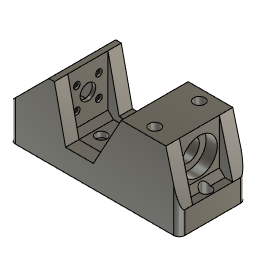
Stepper Motor Mount Mk4 Long v11 (Autodesk Fusion 360 design; units mm, degrees)
Autodesk Fusion 360 part; units mm, degrees
sketch "Sketch1" plane through (0, 0, 0) normal (0, 0, 1) x (1, 0, 0)
  line L0 (0, 0) -> (152, 0)
  line L1 (152, 0) -> (152, 60)
  line L2 (152, 60) -> (0, 60)
  line L3 (0, 60) -> (0, 0)
  dimension "d1" = 152
  dimension "d2" = 60
  constraint horizontal L0
  constraint vertical L1
  constraint horizontal L2
  constraint vertical L3
  constraint coincident L0.start L3.end
  measures "d1" distance of L0.start L0.end
  measures "d2" distance of L0.start L2.end
extrude "Extrude1" add sketch "Sketch1" along normal blind 10
sketch "Sketch2" plane through (0, 0, 10) normal (0, 0, 1) x (-1, 0, 0)
  line L0 (0, -60) -> (0, 0)
  line L1 (0, 0) -> (-152, 0)
  line L2 (-152, 0) -> (-152, -60)
  line L3 (-152, -60) -> (0, -60)
  line L4 (-35, -60) -> (-40, -60)
  line L5 (-40, -60) -> (-40, 0)
  line L6 (-40, 0) -> (-35, 0)
  line L7 (-35, 0) -> (-35, -60)
  line L8 (-140, -60) -> (-100, -60)
  line L9 (-100, -60) -> (-100, 0)
  line L10 (-100, 0) -> (-140, 0)
  line L11 (-140, 0) -> (-140, -60)
  dimension "d5" = 5
  dimension "d6" = 35
  dimension "d25" = 40
  dimension "d91" = 12
  constraint horizontal L4
  constraint vertical L5
  constraint horizontal L6
  constraint vertical L7
  constraint coincident L3 L4.start
  constraint horizontal L8
  constraint vertical L9
  constraint horizontal L10
  constraint vertical L11
  constraint coincident L1 L9.end
  constraint collinear L3 L8
  measures "d5" distance of L4.start L4.end
  measures "d6" distance of L0 L7
  measures "d25" distance of L9 L11
  measures "d91" distance of L2 L11
extrude "Extrude2" add sketch "Sketch2" along normal blind 56 contours L1 L3 L4 L5 L6 L7 | L1 L3 L8 L9 L10 L11
sketch "Sketch3" plane through (40, 0, 0) normal (1, 0, 0) x (0, 1, 0)
  line L0 (0, 10) -> (60, 10)
  line L1 (60, 10) -> (60, 66)
  line L2 (60, 66) -> (0, 66)
  line L3 (0, 66) -> (0, 10)
  circle A0 centre (30, 43) radius 14 construction
  circle A1 centre (20.1005, 52.8995) radius 1.6
  circle A2 centre (39.8995, 52.8995) radius 1.6
  circle A3 centre (20.1005, 33.1005) radius 1.6
  circle A4 centre (39.8995, 33.1005) radius 1.6
  line L4 (30, 43) -> (39.8995, 33.1005) construction
  line L5 (30, 43) -> (45, 43) construction
  line L6 (30, 43) -> (20.1005, 33.1005) construction
  line L7 (30, 43) -> (45, 43) construction
  line L8 (30, 43) -> (20.1005, 52.8995) construction
  line L9 (30, 43) -> (45, 43) construction
  line L10 (30, 43) -> (39.8995, 52.8995) construction
  line L11 (30, 43) -> (45, 43) construction
  circle A5 centre (30, 43) radius 7
  dimension "d9" = 28
  dimension "d10" = 30
  dimension "d11" = 3.2
  dimension "d12" = 3.2
  dimension "d13" = 3.2
  dimension "d14" = 3.2
  dimension "d17" = 33
  dimension "d18" = 45
  dimension "d19" = 135
  dimension "d20" = 135
  dimension "d21" = 45
  dimension "d24" = 14
  constraint coincident A0 A1.centre
  constraint coincident A0 A2.centre
  constraint coincident A0 A3.centre
  constraint coincident A0 A4.centre
  constraint horizontal L5
  constraint coincident A0.centre L4.start
  constraint horizontal L7
  constraint horizontal L9
  constraint horizontal L11
  constraint coincident A4.centre L4.end
  constraint coincident A3.centre L6.end
  constraint coincident A1.centre L8.end
  constraint coincident A2.centre L10.end
  measures "d9" diameter of A0
  measures "d10" distance of L1 A0.centre
  measures "d11" diameter of A1
  measures "d12" diameter of A2
  measures "d13" diameter of A3
  measures "d14" diameter of A4
  measures "d17" distance of L0 A0.centre
  measures "d18" angle of L4 L5
  measures "d19" angle of L6 L7
  measures "d20" angle of L8 L9
  measures "d21" angle of L10 L11
  measures "d24" diameter of A5
extrude "Extrude3" cut sketch "Sketch3" against normal blind 5 contours A1 | A2 | A3 | A4 | A5
sketch "Sketch16" plane through (40, 0, 0) normal (1, 0, 0) x (0, 1, 0)
  circle A0 centre (39.8995, 33.1005) radius 1.6
  circle A1 centre (39.8995, 52.8995) radius 1.6
  circle A2 centre (20.1005, 33.1005) radius 1.6
  circle A3 centre (20.1005, 52.8995) radius 1.6
  circle A4 centre (30, 43) radius 7
  line L0 (0, 10) -> (60, 10)
  line L1 (60, 10) -> (60, 66)
  line L2 (60, 66) -> (0, 66)
  line L3 (0, 66) -> (0, 10)
  circle A5 centre (39.8995, 52.8995) radius 3
  circle A6 centre (39.8995, 33.1005) radius 3
  circle A7 centre (20.1005, 52.8995) radius 3
  circle A8 centre (20.1005, 33.1005) radius 3
  dimension "d132" = 6
  dimension "d133" = 6
  dimension "d134" = 6
  dimension "d135" = 6
  constraint concentric A1 A5
  constraint concentric A0 A6
  constraint concentric A3 A7
  constraint concentric A2 A8
  measures "d132" diameter of A5
  measures "d133" diameter of A6
  measures "d134" diameter of A7
  measures "d135" diameter of A8
extrude "Extrude17" cut sketch "Sketch16" against normal blind 2 contours A5 | A6 | A7 | A8
sketch "Sketch4" plane through (100, 0, 0) normal (-1, 0, 0) x (0, -1, 0)
  line L0 (-60, 10) -> (0, 10)
  line L1 (0, 10) -> (0, 66)
  line L2 (0, 66) -> (-60, 66)
  line L3 (-60, 66) -> (-60, 10)
  circle A0 centre (-30, 43) radius 16.1
  dimension "d26" = 32.2
  dimension "d27" = 30
  dimension "d28" = 33
  measures "d26" diameter of A0
  measures "d27" distance of L1 A0.centre
  measures "d28" distance of L0 A0.centre
extrude "Extrude4" cut sketch "Sketch4" against normal blind 10 contours A0
sketch "Sketch12" plane through (140, 0, 0) normal (1, 0, 0) x (0, 1, 0)
  line L0 (0, 10) -> (60, 10)
  line L1 (60, 10) -> (60, 66)
  line L2 (60, 66) -> (0, 66)
  line L3 (0, 66) -> (0, 10)
  circle A0 centre (30, 43) radius 16.1
  line L4 (0, 10) -> (60, 10)
  dimension "d92" = 32.2
  dimension "d93" = 33
  dimension "d94" = 30
  measures "d92" diameter of A0
  measures "d93" distance of A0.centre L4
  measures "d94" distance of L3 A0.centre
extrude "Extrude12" cut sketch "Sketch12" against normal blind 10 contours A0
sketch "Sketch5" plane through (110, 0, 0) normal (-1, 0, 0) x (0, -1, 0)
  circle A0 centre (-30, 43) radius 16.1
  circle A1 centre (-30, 43) radius 10
  dimension "d31" = 20
  constraint concentric A0 A1
  measures "d31" diameter of A1
extrude "Extrude5" cut sketch "Sketch5" against normal blind 20 contours A1
sketch "Sketch6" plane through (0, 0, 10) normal (0, 0, 1) x (-1, 0, 0)
  line L0 (-100, 0) -> (-100, -60)
  line L1 (-100, -60) -> (-40, -60)
  line L2 (-40, -60) -> (-40, 0)
  line L3 (-40, 0) -> (-100, 0)
  line L4 (-35, 0) -> (-35, -60)
  line L5 (-35, -60) -> (0, -60)
  line L6 (0, -60) -> (0, 0)
  line L7 (0, 0) -> (-35, 0)
  line L8 (-40, -60) -> (-100, -60)
  line L9 (-100, -60) -> (-100, -48)
  line L10 (-100, -48) -> (-40, -48)
  line L11 (-40, -48) -> (-40, -60)
  line L12 (-40, 0) -> (-100, 0)
  line L13 (-100, 0) -> (-100, -12)
  line L14 (-100, -12) -> (-40, -12)
  line L15 (-40, -12) -> (-40, 0)
  line L16 (-35, -60) -> (0, -60)
  line L17 (0, -60) -> (0, -52)
  line L18 (0, -52) -> (-35, -52)
  line L19 (-35, -52) -> (-35, -60)
  line L20 (-35, 0) -> (0, 0)
  line L21 (0, 0) -> (0, -8)
  line L22 (0, -8) -> (-35, -8)
  line L23 (-35, -8) -> (-35, 0)
  line L24 (-140, -60) -> (-140, 0)
  line L25 (-140, 0) -> (-152, 0)
  line L26 (-152, 0) -> (-152, -60)
  line L27 (-152, -60) -> (-140, -60)
  line L28 (-140, -60) -> (-152, -60)
  line L29 (-152, -60) -> (-152, -48)
  line L30 (-152, -48) -> (-140, -48)
  line L31 (-140, -48) -> (-140, -60)
  line L32 (-140, 0) -> (-152, 0)
  line L33 (-152, 0) -> (-152, -12)
  line L34 (-152, -12) -> (-140, -12)
  line L35 (-140, -12) -> (-140, 0)
  dimension "d34" = 12
  dimension "d35" = 12
  dimension "d128" = 12
  dimension "d129" = 12
  dimension "d130" = 8
  dimension "d168" = 8
  constraint horizontal L8
  constraint vertical L9
  constraint horizontal L10
  constraint vertical L11
  constraint coincident L1.end L2.start
  constraint horizontal L12
  constraint vertical L13
  constraint horizontal L14
  constraint vertical L15
  constraint coincident L2.end L3.start
  constraint horizontal L16
  constraint vertical L17
  constraint horizontal L18
  constraint vertical L19
  constraint coincident L6 L17.end
  constraint coincident L4.end L5.start
  constraint horizontal L20
  constraint vertical L21
  constraint horizontal L22
  constraint vertical L23
  constraint coincident L6 L21.end
  constraint coincident L4.start L7.end
  constraint collinear L0 L13
  constraint collinear L0 L9
  constraint horizontal L28
  constraint vertical L29
  constraint horizontal L30
  constraint vertical L31
  constraint coincident L26 L29.end
  constraint coincident L24.start L27.end
  constraint horizontal L32
  constraint vertical L33
  constraint horizontal L34
  constraint vertical L35
  constraint coincident L26 L33.end
  constraint coincident L24.end L25.start
  measures "d34" distance of L1.end L10.end
  measures "d35" distance of L2.end L14.end
  measures "d128" distance of L28 L30
  measures "d129" distance of L32 L34
  measures "d130" distance of L20 L22
  measures "d168" distance of L16 L18
extrude "Extrude6" add sketch "Sketch6" along normal blind 56 contours L0 L2 L3 L12 L13 L14 L15 | L0 L1 L2 L8 L9 L10 L11 | L4 L6 L7 L20 L21 L22 L23 | L4 L5 L6 L16 L17 L18 L19 | L24 L26 L27 L28 L29 L30 L31 | L24 L25 L26 L32 L33 L34 L35
chamfer "Chamfer1" distance 35 angle 45 2 edges at (0, 4, 66) (0, 56, 66)
sketch "Sketch7" plane through (0, 0, 0) normal (0, -1, 0) x (1, 0, 0)
  line L0 (35, 66) -> (0, 31)
  line L1 (0, 31) -> (0, 0)
  line L2 (0, 0) -> (152, 0)
  line L3 (152, 0) -> (152, 66)
  line L4 (152, 66) -> (35, 66)
  line L5 (40, 66) -> (100, 66)
  line L6 (100, 66) -> (100, 10)
  line L7 (100, 10) -> (40, 10)
  line L8 (40, 10) -> (40, 66)
  line L9 (40, 20) -> (100, 20)
  line L10 (40, 20) -> (40, 66)
  line L11 (100, 10) -> (100, 66)
  line L12 (152, 66) -> (140, 66)
  line L13 (140, 66) -> (140, 20)
  line L14 (140, 20) -> (152, 20)
  line L15 (152, 20) -> (152, 66)
  point P0 (40, 66)
  point P1 (140, 66)
  dimension "d41" = 56
  dimension "d44" = 10
  constraint horizontal L5
  constraint vertical L6
  constraint horizontal L7
  constraint vertical L8
  constraint coincident L4 P0
  constraint coincident L8 L9.start
  constraint coincident L6 L9.end
  constraint perpendicular L6 L9
  constraint vertical L10
  constraint collinear L6 L11
  constraint coincident P0 L5.start
  constraint horizontal L12
  constraint vertical L13
  constraint horizontal L14
  constraint vertical L15
  constraint coincident L3.end L4.start
  constraint coincident L13 P1
  constraint collinear L9 L14
  measures "d41" distance of L5 L7
  measures "d44" distance of L7 L9
extrude "Extrude7" cut sketch "Sketch7" against normal blind 60 contours L4 L5 L6 L8 L9 L10 L11 | L3 L4 L12 L13 L14 L15
chamfer "Chamfer2" distance 46 distance2 10 2 edges at (40, 6, 20) (40, 54, 20) measured on face at (40, 27.2002, 16.8341) measured on face at (40, 27.2002, 16.8341)
chamfer "Chamfer3" distance 25 distance2 46 2 edges at (100, 54, 20) (100, 6, 20) measured on face at (66.6653, 52, 20) measured on face at (66.6653, 4, 20)
sketch "Sketch8" plane through (0, 0, 10) normal (0, 0, 1) x (-1, 0, 0)
  circle A0 centre (-64, -30) radius 2.6
  circle A1 centre (-76, -30) radius 2.6
  circle A2 centre (-88, -30) radius 2.6
  line L0 (-40, -12) -> (-100, -12)
  line L1 (-100, -12) -> (-100, -48)
  line L2 (-100, -48) -> (-40, -48)
  line L3 (-40, -48) -> (-40, -12)
  circle A3 centre (-22, -30) radius 2.6
  circle A4 centre (-8, -30) radius 2.6
  line L4 (0, -52) -> (0, -8)
  circle A5 centre (-146, -30) radius 2.6
  line L5 (-152, 0) -> (-140, 0)
  line L6 (-152, -12) -> (-152, -48)
  circle A6 centre (-52, -30) radius 2.6
  line L7 (-40, 0) -> (-50, 0)
  dimension "d48" = 5.2
  dimension "d49" = 5.2
  dimension "d50" = 5.2
  dimension "d58" = 12
  dimension "d59" = 12
  dimension "d71" = 5.2
  dimension "d73" = 5.2
  dimension "d78" = 8
  dimension "d83" = 12
  dimension "d118" = 5.2
  dimension "d119" = 30
  dimension "d120" = 6
  dimension "d138" = 14
  dimension "d139" = 5.2
  dimension "d140" = 12
  dimension "d169" = 30
  dimension "d170" = 30
  dimension "d171" = 30
  dimension "d172" = 30
  dimension "d173" = 30
  dimension "d174" = 30
  measures "d48" diameter of A0
  measures "d49" diameter of A1
  measures "d50" diameter of A2
  measures "d58" distance of A0.centre A1.centre
  measures "d59" distance of A1.centre A2.centre
  measures "d71" diameter of A3
  measures "d73" diameter of A4
  measures "d78" distance of A4.centre L4
  measures "d83" distance of A2.centre L1
  measures "d118" diameter of A5
  measures "d119" distance of A5.centre L5
  measures "d120" distance of A5.centre L6
  measures "d138" distance of A3.centre A4.centre
  measures "d139" diameter of A6
  measures "d140" distance of A0.centre A6.centre
  measures "d169" distance of A6.centre L7
  measures "d170" distance of A0.centre L7
  measures "d171" distance of A1.centre L7
  measures "d172" distance of A2.centre L7
  measures "d173" distance of A4.centre L7
  measures "d174" distance of A3.centre L7
extrude "Extrude8" cut sketch "Sketch8" against normal blind 10 contours A0 | A1 | A2 | A3 | A4 | A5 | A6
sketch "Sketch17" plane through (0, 0, 10) normal (0, 0, 1) x (-1, 0, 0)
  circle A0 centre (-88, -30) radius 2.6
  circle A1 centre (-76, -30) radius 2.6
  circle A2 centre (-64, -30) radius 2.6
  circle A3 centre (-52, -30) radius 2.6
  line L0 (-100, -48) -> (-40, -48)
  line L1 (-40, -48) -> (-40, -12)
  line L2 (-40, -12) -> (-100, -12)
  line L3 (-100, -12) -> (-100, -48)
  circle A4 centre (-8, -30) radius 2.6
  circle A5 centre (-22, -30) radius 2.6
  line L4 (-35, -52) -> (0, -52)
  line L5 (0, -52) -> (0, -8)
  line L6 (0, -8) -> (-35, -8)
  line L7 (-35, -8) -> (-35, -52)
  circle A6 centre (-146, -30) radius 2.6
  line L8 (-152, -48) -> (-140, -48)
  line L9 (-140, -48) -> (-140, -12)
  line L10 (-140, -12) -> (-152, -12)
  line L11 (-152, -12) -> (-152, -48)
  circle A7 centre (-8, -30) radius 5
  circle A8 centre (-22, -30) radius 5
  circle A9 centre (-52, -30) radius 5
  circle A10 centre (-64, -30) radius 5
  circle A11 centre (-76, -30) radius 5
  circle A12 centre (-88, -30) radius 5
  circle A13 centre (-146, -30) radius 5
  dimension "d141" = 10
  dimension "d142" = 10
  dimension "d143" = 10
  dimension "d144" = 10
  dimension "d145" = 10
  dimension "d146" = 10
  dimension "d147" = 10
  constraint concentric A4 A7
  constraint concentric A5 A8
  constraint concentric A3 A9
  constraint concentric A2 A10
  constraint concentric A1 A11
  constraint concentric A0 A12
  constraint concentric A6 A13
  measures "d141" diameter of A7
  measures "d142" diameter of A8
  measures "d143" diameter of A9
  measures "d144" diameter of A10
  measures "d145" diameter of A11
  measures "d146" diameter of A12
  measures "d147" diameter of A13
extrude "Extrude18" add sketch "Sketch17" along normal blind 5 contours L0 L1 L2 L3 | L4 L5 L6 L7 | L8 L9 L10 L11
chamfer "Chamfer6" distance 46 distance2 12 2 edges at (140, 6, 20) (140, 54, 20) measured on face at (140, 55.3667, 43) measured on face at (140, 55.3667, 43)
fillet "Fillet1" radius 5 4 edges at (0, 0, 15.5) (0, 60, 15.5) (152, 0, 10) (152, 60, 10)
extrude "Extrude19" add 1 faces at (145.8754, 43.662, 15) along direction (0, 0, 1) blind 5
chamfer "Chamfer4" distance 5 angle 45 4 edges at (140, 30, 20) (100, 30, 15) (40, 30, 15) (35, 30, 15)
sketch "Sketch10" plane through (35, 0, 0) normal (-1, 0, 0) x (0, -1, 0)
  line L0 (-8, 20) -> (-8, 66)
  line L1 (-52, 66) -> (-52, 20)
  circle A0 centre (-30, 43) radius 11.5
  circle A1 centre (-20.1005, 33.1005) radius 1.6
  circle A2 centre (-39.8995, 33.1005) radius 1.6
  circle A3 centre (-39.8995, 52.8995) radius 1.6
  circle A4 centre (-20.1005, 52.8995) radius 1.6
  circle A5 centre (-30, 43) radius 7
  line L2 (-8, 66) -> (-52, 66)
  line L3 (-52, 20) -> (-8, 20)
  dimension "d79" = 23
  measures "d79" diameter of A0
extrude "Extrude10" cut sketch "Sketch10" against normal blind 2 contours A0 | A5
sketch "Sketch19" plane through (0, 0, 66) normal (0, 0, 1) x (-1, 0, 0)
  line L0 (-100, -60) -> (-100, -48)
  line L1 (-100, -48) -> (-100, -12)
  line L2 (-100, -12) -> (-100, 0)
  line L3 (-100, 0) -> (-140, 0)
  line L4 (-140, 0) -> (-140, -12)
  line L5 (-140, -12) -> (-140, -48)
  line L6 (-140, -48) -> (-140, -60)
  line L7 (-140, -60) -> (-100, -60)
  circle A0 centre (-120, -50) radius 2.6
  circle A1 centre (-120, -10) radius 2.6
  dimension "d155" = 5.2
  dimension "d156" = 5.2
  dimension "d157" = 10
  dimension "d158" = 10
  dimension "d161" = 20
  dimension "d162" = 20
  measures "d155" diameter of A0
  measures "d156" diameter of A1
  measures "d157" distance of L3 A1.centre
  measures "d158" distance of L7 A0.centre
  measures "d161" distance of L0 A0.centre
  measures "d162" distance of L2 A1.centre
extrude "Extrude20" cut sketch "Sketch19" against normal blind 66 contours A0 | A1
sketch "Sketch20" plane through (0, 0, 66) normal (0, 0, 1) x (-1, 0, 0)
  circle A0 centre (-120, -50) radius 2.6
  circle A1 centre (-120, -10) radius 2.6
  line L0 (-100, -60) -> (-100, -48)
  line L1 (-100, -48) -> (-100, -12)
  line L2 (-100, -12) -> (-100, 0)
  line L3 (-100, 0) -> (-140, 0)
  line L4 (-140, 0) -> (-140, -12)
  line L5 (-140, -12) -> (-140, -48)
  line L6 (-140, -48) -> (-140, -60)
  line L7 (-140, -60) -> (-100, -60)
  circle A2 centre (-120, -50) radius 5
  circle A3 centre (-120, -10) radius 5
  dimension "d164" = 10
  dimension "d165" = 10
  constraint concentric A0 A2
  constraint concentric A1 A3
  measures "d164" diameter of A2
  measures "d165" diameter of A3
extrude "Extrude21" cut sketch "Sketch20" against normal blind 19 contours A2 | A3
